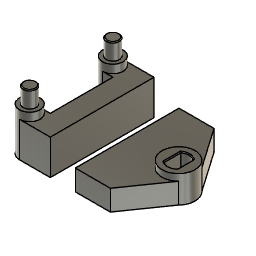
SensorMountFinished v1 (Autodesk Fusion 360 design; units mm, degrees)
Autodesk Fusion 360 part; units mm, degrees
note: some values were not read from the file. Chosen so that the rebuilt part matches the saved one: which bodies a step acts on. Set by a fixed rule: which sketch regions a step uses.
sketch "Sketch1" plane through (0, 0, 0) normal (0, 0, 1) x (1, 0, 0)
  circle A0 centre (4.925, 7.5) radius 2.5
  circle A1 centre (25.0889, 7.4888) radius 2.4889
  circle A2 centre (4.925, 7.5) radius 1.575
  circle A3 centre (25.0889, 7.4888) radius 1.575
  line L0 (27.5778, 7.4888) -> (27.5778, 0)
  line L1 (2.425, 7.5) -> (2.425, 0)
  line L2 (2.425, 0) -> (27.5778, 0)
  line L3 (7.425, 5) -> (22.6, 5)
  line L4 (22.6, 7.4888) -> (22.6, 5)
  line L5 (7.425, 5) -> (7.425, 7.5)
  dimension "d78" = 3.15
  dimension "d79" = 7.5
  constraint concentric A0 A2
  constraint concentric A1 A3
  constraint coincident A1 L0.start
  constraint tangent A1 L0
  constraint coincident A0 L1.start
  constraint tangent A0 L1
  constraint perpendicular L0 L2
  constraint coincident A1 L4.start
  constraint coincident A0 L5.end
  measures "d78" diameter of A2
  measures "d79" distance of A0.centre L2
extrude "Extrude9" add sketch "Sketch1" along normal blind 14.5 contours A2 | A3 makes body 1 at (6.498, 7.4215, 9.6667) makes body 2 at (26.6619, 7.4103, 9.6667)
extrude "Extrude10" add sketch "Sketch1" along normal blind 10.5 contours A0 | A1 bodies 1 2
extrude "Extrude11" add sketch "Sketch1" along normal blind 8.5 contours A0 A1 L0 L1 L2 L3 L4 L5 bodies 1 2
fillet "Fillet2" radius 0.2 2 edges at (23.6205, 6.9193, 14.5) (3.4566, 6.9305, 14.5) on bodies 1 2
sketch "Sketch4" plane through (0, 0, 0) normal (0, 0, 1) x (1, 0, 0)
  line L0 (0, 0) -> (25.1528, 0)
  line L1 (25.1528, 0) -> (25.1528, 8.5)
  line L2 (25.1528, 8.5) -> (0, 8.5)
  line L3 (0, 8.5) -> (0, 0)
  circle A0 centre (12.5771, 12.465) radius 2.5
  circle A1 centre (12.5771, 12.465) radius 4
  line L4 (12.5771, 11) -> (10.5513, 11)
  line L5 (12.5771, 14.08) -> (10.6688, 14.08)
  line L6 (9.7482, 15.2929) -> (0, 8.5)
  line L7 (15.4055, 15.2934) -> (25.1528, 8.5)
  line L8 (14.6029, 11) -> (10.5513, 11)
  line L9 (14.4854, 14.08) -> (10.6688, 14.08)
  dimension "d42" = 25.1528
  dimension "d43" = 8.5
  dimension "d73" = 3.08
  constraint horizontal L0
  constraint vertical L1
  constraint horizontal L2
  constraint vertical L3
  constraint coincident L0.start L3.end
  constraint concentric A0 A1
  constraint coincident A0 L8.start
  constraint coincident A0 L4.end
  constraint coincident A0 L9.start
  constraint coincident A0 L5.end
  constraint coincident A1 L7.start
  constraint coincident A1 L6.start
  constraint parallel L4 L8
  constraint parallel L5 L9
  measures "d42" distance of L0.start L0.end
  measures "d43" distance of L0.start L2.end
  measures "d73" distance of L8 L9
extrude "Extrude12" add sketch "Sketch4" along normal blind 5 separate body contours L0 L1 L2 L3 A1 | L2 A1 L6 | L2 A1 L7 makes body 3
extrude "Extrude13" add sketch "Sketch4" along normal blind 5 contours L2 A1 picked at (12.5166, 8.9905) bodies 3
extrude "Extrude14" add sketch "Sketch4" along normal blind 5 contours L2 A1 | A0 L5 L9 | A0 L4 L8 picked at (12.5183, 8.4896) bodies 3
extrude "Extrude15" add sketch "Sketch4" along normal blind 0.5 contours A0 L4 L5 L8 L9 bodies 3
extrude "Extrude16" cut sketch "Sketch4" along normal blind 7 contours A0 L5 L9 | A0 L4 L8 bodies 3
extrude "Extrude17" add sketch "Sketch4" along normal blind 7 contours A0 L5 L9 | A0 L4 L8 bodies 3
extrude "Extrude18" cut sketch "Sketch4" along normal blind 7 contours L2 A1 picked at (12.5166, 8.9905) bodies 3 makes body 4 at (12.4006, 2.8333, 0)
extrude "Extrude19" add sketch "Sketch4" along normal blind 7 contours L2 A1 picked at (12.5166, 8.9905) bodies 3 4
extrude "Extrude20" cut sketch "Sketch4" along normal blind 7 contours L2 A1 picked at (12.5183, 8.4896) bodies 3
extrude "Extrude21" add sketch "Sketch4" along normal blind 7 contours L2 A1 picked at (12.5183, 8.4896) bodies 3
extrude "Extrude22" cut 1 faces at (12.6001, 10.1552, 7) along direction (0, 0, -1) blind 0.4 on bodies 3 bodies 3
fillet "Fillet3" radius 0.2 4 edges at (15.0753, 12.5603, 6.6) (12.5771, 14.08, 6.6) (10.0789, 12.5603, 6.6) (12.5771, 11, 6.6) on bodies 3
move_body "Move1" bodies 1 to x (0, 1, 0) y (-1, 0, 0) z (0, 0, 1) at (-0.9986, -15.0014, 0)
move_body "Move2" bodies 3 to x (0, -1, 0) y (1, 0, 0) z (0, 0, 1) at (0.0371, 13.1171, 0)
move_body "Move3" bodies 3 to x (1, 0, 0) y (0, 1, 0) z (0, 0, 1) at (5, 0, 0)
move_body "Move4" bodies 1 to x (1, 0, 0) y (0, 1, 0) z (0, 0, 1) at (0, 0.5, 0)
extrude "Extrude5" [rolled back] along distance 0.5 taper angle 0
extrude "Extrude6" [rolled back] along distance 0.5 taper angle 0
extrude "Extrude7" [rolled back] along distance -0.5 taper angle 0
extrude "Extrude8" [rolled back] along distance -0.5 taper angle 0
